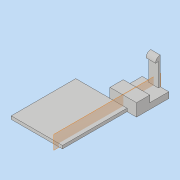
# Autodesk Inventor part: arduinomount
Saved by Autodesk Inventor 2017 (Build 210142000, 142)
## iProperties
Created: 2017-02-25
Part Number: arduinomount
Material: Generic
Document SubType Name: Modeling
Designer: Joshua Yuan
Density: 1 g/cm^3
Appearance: Default
Author: Joshua Yuan
Autodesk Inventor part; units mm, degrees
ref_plane "YZ Plane" through (0, 0, 0) normal (1, 0, 0) x (0, 1, 0)
ref_plane "XZ Plane" through (0, 0, 0) normal (0, 1, 0) x (-1, 0, 0)
ref_plane "XY Plane" through (0, 0, 0) normal (0, 0, 1) x (1, 0, 0)
sketch "Sketch1" plane through (0, 0, 0) normal (0, 1, 0) x (-1, 0, 0)
  line L0 (15.8213, 9.9209) -> (-38.1787, 9.9209)
  line L1 (-38.1787, 9.9209) -> (-38.1787, -58.0791)
  line L2 (-38.1787, -58.0791) -> (15.8213, -58.0791)
  line L3 (15.8213, -58.0791) -> (15.8213, 9.9209)
  line L4 (-20.1787, -58.0791) -> (-48.1787, -58.0791)
  line L5 (-48.1787, -58.0791) -> (-48.1787, -92.0791)
  line L6 (-48.1787, -92.0791) -> (-20.1787, -92.0791)
  line L7 (-20.1787, -92.0791) -> (-20.1787, -58.0791)
  point P0 (0, 0)
  dimension "d0" = 54
  dimension "d1" = 68
  dimension "d2" = 28
  dimension "d3" = 10
  dimension "d4" = 34
  constraints: 16 end point, 4 parallel, 2 horizontal, 2 perpendicular, 1 point on line
  measures "d0" distance of L0.start L0.end
  measures "d1" distance of L0.end L1.end
  measures "d2" distance of L5.end L6.end
  measures "d3" distance between parallel lines of L1 L5
  measures "d4" distance of L4.end L5.end
extrude "Extrusion1" add sketch "Sketch1" against normal blind 3.175
sketch "Sketch2" plane through (0, 0, 0) normal (0, 1, 0) x (1, 0, 0)
  line L0 (20.1787, 92.0791) -> (20.1787, 58.0791) projected
  line L1 (48.1787, 58.0791) -> (48.1787, 92.0791) projected
  line L2 (20.1787, 92.0791) -> (48.1787, 92.0791)
  line L3 (48.1787, 92.0791) -> (48.1787, 72.0791)
  line L4 (48.1787, 72.0791) -> (20.1787, 72.0791)
  line L5 (20.1787, 72.0791) -> (20.1787, 92.0791)
  line L6 (38.1787, 58.0791) -> (48.1787, 58.0791) projected
  point P0 (0, 0)
  dimension "d7" = 14
  constraints: 8 end point, 2 parallel, 1 horizontal, 1 perpendicular, 1 point on line
  measures "d7" distance between parallel lines of L6 L4
extrude "Extrusion2" add sketch "Sketch2" along normal blind 3
sketch "Sketch3" plane through (0, 0, 0) normal (0, 1, 0) x (1, 0, 0)
  line L0 (48.1787, 72.0791) -> (20.1787, 72.0791) projected
  line L1 (48.1787, 92.0791) -> (48.1787, 58.0791) projected
  line L2 (20.1787, 72.0791) -> (48.1787, 72.0791)
  line L3 (48.1787, 72.0791) -> (48.1787, 58.0791)
  line L4 (48.1787, 58.0791) -> (20.1787, 58.0791)
  line L5 (20.1787, 58.0791) -> (20.1787, 72.0791)
  point P0 (0, 0)
  constraints: 8 end point, 2 parallel, 1 horizontal, 1 perpendicular
extrude "Extrusion3" add sketch "Sketch3" along normal blind 10
ref_plane "Work Plane1" through (34.1787, -3.175, -58.0791) normal (1, 0, 0) x (0, 0, -1)
sketch "Sketch4" plane through (34.1787, -3.175, -58.0791) normal (1, 0, 0) x (0, 0, -1)
  line L0 (29, 30.175) -> (32, 30.175)
  line L1 (32, 30.175) -> (32, 6.175)
  line L2 (34, 6.175) -> (14, 6.175) projected
  line L3 (34, 6.175) -> (34, 35.175)
  arc A0 (34, 35.175) -> (29, 30.175) centre (34, 30.175) ccw
  point P0 (-58.0791, 3.175)
  dimension "d12" = 2
  dimension "d13" = 29
  dimension "d14" = 24
  dimension "d15" = 3
  constraints: 6 end point, 2 point on circle, 2 point on line, 1 centre point, 1 horizontal, 1 perpendicular, 1 vertical
  measures "d12" distance between parallel lines of L3 L1
  measures "d13" distance of L2.start L3.end
  measures "d14" distance of L0.end L1.end
  measures "d15" distance of L0.start L0.end
extrude "Extrusion4" add sketch "Sketch4" along normal mid plane 10
body "Solid1"
